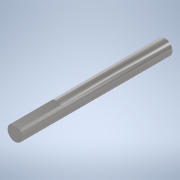
# Autodesk Inventor part: Shaft
Saved by Autodesk Inventor 2022 (Build 260153000, 153)
## iProperties
Created: 2022-09-16
Part Number: Shaft
Material: Stainless Steel
Document SubType Name: Modeling
Designer: Nathan Cai
Density: 8 g/cm^3
Appearance: Semi-Polished
Author: Nathan Cai
Autodesk Inventor part; units mm, degrees
ref_plane "YZ Plane" through (0, 0, 0) normal (1, 0, 0) x (0, 1, 0)
ref_plane "XZ Plane" through (0, 0, 0) normal (0, 1, 0) x (-1, 0, 0)
ref_plane "XY Plane" through (0, 0, 0) normal (0, 0, 1) x (1, 0, 0)
sketch "Sketch1" plane through (0, 0, 0) normal (0, 0, 1) x (1, 0, 0)
  circle A0 centre (0, 0) radius 5
  dimension "d0" = 10
  constraints: 1 centre point, 1 coincident
  measures "d0" diameter of A0
extrude "Extrusion1" add sketch "Sketch1" along normal blind 101
sketch "Sketch2" plane through (0, 0, 101) normal (0, 0, 1) x (1, 0, 0)
  circle A0 centre (0, 0) radius 5
  circle A1 centre (0, 0) radius 5 projected
  line L0 (-5, 0) -> (0, 0) construction
  line L1 (-3, 4) -> (3, 4)
  dimension "d3" = 10
  dimension "d4" = 4
  constraints: 4 end point, 3 point on circle, 2 horizontal, 1 centre point, 1 coincident, 1 parallel
  measures "d3" diameter of A0
  measures "d4" distance from line of L1 point (0, 0)
extrude "Extrusion2" cut sketch "Sketch2" against normal blind 28 contours L1 A0 picked at (-0.6933, 4.1823)
body "Solid1"
